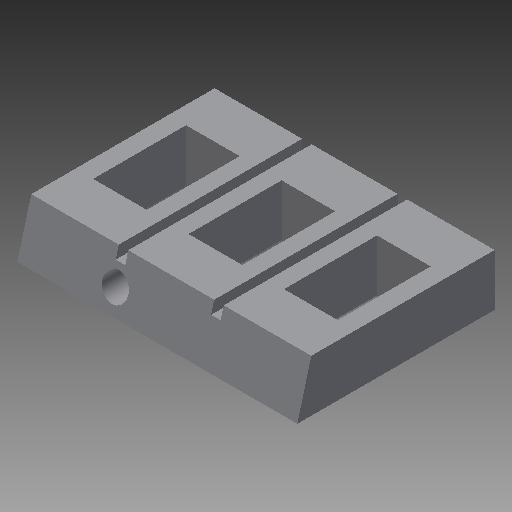
# Autodesk Inventor part: nzm1_3p_p2
Saved by Autodesk Inventor 2019.3 (Build 233278000, 278)
## iProperties
Category: PARTsolutions
Company: MOELLER
Created: 2018-10-25
Part Number: nzm1_3p_p2
Material: Generic
Catalog Web Link: www.cadenas.de
Description: Leistungsschalter 3p_p2-Leistungsschalter 3p
Vendor: MOELLER
Document SubType Name: Modeling
Designer: psadmin
Manufacturer: MOELLER
Mass: 58.865 g
Surface Area: 187.652 cm^2
Volume: 58.865 cm^3
Density: 1 g/cm^3
Appearance: PSOLRGB-192-192-192
PSOL_IDENT_0: {$CADENAS_DATA\23d-libs\moeller\circuit_breaker\parts\nzm1_3p_p2.prj},178 {VTYP=3D},{NB=nzm1_3p_p2},
PSOL_IDENT_1: {LINA=nzm1_3p_p2},{NN=Leistungsschalter 3p_p2},{DATE=05.10.2018 14:14:16},{GEOMDATE=14.05.2018 10:43
PSOL_IDENT_2: :05},{VERSION=},{LINEID=310},{WBVAR=},{WBNUMERIC=}  {NB=nzm1_3p_p2},{LINA=nzm1_3p_p2},{KT=DUMMY},{BM
PSOL_IDENT_3: ENB=nzm1_3p_p2},{EPLAN=}
NN: Leistungsschalter 3p_p2
NT: Leistungsschalter 3p
NB: nzm1_3p_p2
NBSYN: $BMENB.
LINA: nzm1_3p_p2
BMENB: nzm1_3p_p2
SUPPLIER: MOELLER
ARTICLENO: nzm1_3p_p2
BOMINFO: nzm1_3p_p2
CREATOR: CADENAS GmbH
Title: nzm1_3p_p2
Author: Cadenas PARTsolutions
Comments: Leistungsschalter 3p
Autodesk Inventor part; units mm, degrees
sketch "Sketch_1" plane through (0, 0, 0) normal (1, 0, 0) x (0, 1, 0)
  line L0 (0, 61.9996) -> (0, 0)
  line L1 (0, 0) -> (16.3, 0)
  line L2 (16.3, 0) -> (16.3, 57.632)
  line L3 (16.3, 57.632) -> (0, 61.9996)
  constraints: 8 end point
extrude "Extrusion1" add sketch "Sketch_1" along normal blind 88
sketch "Sketch_2" plane through (0, 0, 0) normal (0, 0, 1) x (1, 0, 0)
  line L0 (27.5, 20.7) -> (27.5, 12.7)
  line L1 (27.5, 12.7) -> (30.5, 12.7)
  line L2 (30.5, 12.7) -> (30.5, 17.7)
  line L3 (30.5, 17.7) -> (57.5, 17.7)
  line L4 (57.5, 17.7) -> (57.5, 12.7)
  line L5 (57.5, 12.7) -> (60.5, 12.7)
  line L6 (60.5, 12.7) -> (60.5, 20.7)
  line L7 (60.5, 20.7) -> (27.5, 20.7)
  constraints: 16 end point
extrude "Extrusion2" cut sketch "Sketch_2" along normal blind 65
sketch "Sketch_3" plane through (0, 0, 14.55) normal (0, 0, 1) x (1, 0, 0)
  line L0 (5.575, 27) -> (5.575, 0)
  line L1 (5.575, 0) -> (22.425, 0)
  line L2 (22.425, 0) -> (22.425, 22)
  line L3 (22.425, 22) -> (35.575, 22)
  line L4 (35.575, 22) -> (35.575, 0)
  line L5 (35.575, 0) -> (52.425, 0)
  line L6 (52.425, 0) -> (52.425, 22)
  line L7 (52.425, 22) -> (65.575, 22)
  line L8 (65.575, 22) -> (65.575, 0)
  line L9 (65.575, 0) -> (82.425, 0)
  line L10 (82.425, 0) -> (82.425, 27)
  line L11 (82.425, 27) -> (5.575, 27)
  constraints: 24 end point
extrude "Extrusion3" cut sketch "Sketch_3" along normal blind 29.2
sketch "Sketch_5" plane through (29, 0, 0) normal (1, 0, 0) x (0, 0, -1)
  line L0 (0, 6.8) -> (-63, 6.8)
  line L1 (-63, 6.8) -> (-63, 10.9)
  line L2 (-63, 10.9) -> (-40, 10.9)
  line L3 (-40, 10.9) -> (-40, 8.9)
  line L4 (-40, 8.9) -> (0, 8.9)
  line L5 (0, 8.9) -> (0, 6.8)
  line L6 (0, 6.8) -> (-63, 6.8)
  constraints: 14 end point
revolve "Revolution1" cut sketch "Sketch_5" angle 360 about axis through (29, 6.8, 0) along (0, 0, -1)
ref_plane "P2_XY" through (-1, 0, 0) normal (0, -1, 0) x (1, 0, 0)
ref_plane "P2_YZ" through (-1, 0, 0) normal (1, 0, 0) x (0, 0, 1)
ref_plane "P2_ZX" through (-1, 0, 0) normal (0, 0, 1) x (0, -1, 0)
body "Solid1"
